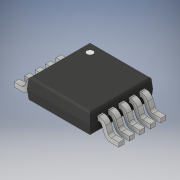
# Autodesk Inventor part: Semiconductor_TSOP-10
Saved by Autodesk Inventor 2017 (Build 210142000, 142)
## iProperties
Created: 2016-07-22
Part Number: Semiconductor_TSOP-10
Material: ABS Plastic
Document SubType Name: Modeling
Designer: Bradley
Density: 1.06 g/cm^3
Appearance: Smooth - Black
Mass: 0.00993513 g
Surface Area: 0.40182 cm^2
Volume: 0.00937276 cm^3
Author: Bradley
Autodesk Inventor part; units mm, degrees
ref_plane "YZ Plane" through (0, 0, 0) normal (1, 0, 0) x (0, 1, 0)
ref_plane "XZ Plane" through (0, 0, 0) normal (0, 1, 0) x (-1, 0, 0)
ref_plane "XY Plane" through (0, 0, 0) normal (0, 0, 1) x (1, 0, 0)
sketch "Sketch1" plane through (0, 0, 0) normal (0, 1, 0) x (-1, 0, 0)
  line L0 (-1.5, 1.5) -> (1.5, 1.5)
  line L1 (1.5, 1.5) -> (1.5, -1.5)
  line L2 (1.5, -1.5) -> (-1.5, -1.5)
  line L3 (-1.5, -1.5) -> (-1.5, 1.5)
  line L4 (-1.5, 1.5) -> (1.5, -1.5) construction
  line L5 (1.5, 1.5) -> (-1.5, -1.5) construction
  point P0 (0, 0)
  dimension "d0" = 3
  dimension "d1" = 3
  constraints: 12 end point, 2 midpoint, 2 parallel, 1 horizontal, 1 perpendicular
  measures "d0" distance of L1.end L2.end
  measures "d1" distance of L0.end L1.end
extrude "Extrusion1" add sketch "Sketch1" along normal blind 0.5 draft -5
sketch "Sketch2" plane through (0, 0, 0) normal (0, -1, 0) x (1, 0, 0)
  line L0 (1.5, 1.5) -> (-1.5, 1.5) projected
  line L1 (1.5, 1.5) -> (-1.5, 1.5) projected
  line L2 (-1.5, 1.5) -> (-1.5, -1.5) projected
  line L3 (-1.5, -1.5) -> (1.5, -1.5) projected
  line L4 (1.5, -1.5) -> (1.5, 1.5) projected
  point P0 (0, 0)
extrude "Extrusion2" add sketch "Sketch2" along normal blind 0.5 draft -5
fillet "Fillet1" radius 0.1 8 edges at (-1.4563, 0.5, 0) (0, 0.5, 1.4563) (0, 0.5, -1.4563) (1.4563, 0.5, 0) (1.4563, -0.5, 0) (0, -0.5, 1.4563) (-1.4563, -0.5, 0) (0, -0.5, -1.4563)
sketch "Sketch3" plane through (0, 0, 0) normal (0, 1, 0) x (-1, 0, 0)
  line L0 (1.5, 1.5) -> (1.5, -1.5) projected
  line L1 (-1.5, 1.5) -> (1.5, 1.5) projected
  line L2 (1.5, 1.125) -> (1.55, 1.125)
  line L3 (1.55, 1.125) -> (1.55, 0.875)
  line L4 (1.55, 0.875) -> (1.5, 0.875)
  line L5 (1.5, 0.875) -> (1.5, 1.125)
  line L6 (-1.5, -1.5) -> (-1.5, 1.5) projected
  line L7 (-1.5, 1.125) -> (-1.55, 1.125)
  line L8 (-1.55, 1.125) -> (-1.55, 0.875)
  line L9 (-1.55, 0.875) -> (-1.5, 0.875)
  line L10 (-1.5, 0.875) -> (-1.5, 1.125)
  line L11 (-1.5, 0.875) -> (1.5, 0.875)
  line L12 (1.5, 0.875) -> (1.5, 1.125)
  line L13 (1.5, 1.125) -> (-1.5, 1.125)
  line L14 (-1.5, 1.125) -> (-1.5, 0.875)
  point P0 (0, 0)
  point P1 (1.5, 1)
  dimension "d7" = 0.25
  dimension "d8" = 1
  dimension "d9" = 0.05
  constraints: 24 end point, 6 parallel, 4 point on line, 3 horizontal, 3 perpendicular, 1 collinear, 1 midpoint
  measures "d7" distance of L2.end L3.end
  measures "d8" vertical distance of point (1.5, 1) point (0, 0)
  measures "d9" distance of L3.end L4.end
extrude "Extrusion3" add sketch "Sketch3" along normal blind 0.2 contours L2 L3 L4 L0 | L0 L11 L6 L13 | L6 L9 L8 L7
sketch "Sketch4" plane through (-1.55, 0, 1.125) normal (0, 0, 1) x (1, 0, 0)
  line L0 (0.0675, 0.2) -> (0.05, 0) projected
  line L1 (0, 0.2) -> (0.0675, 0.2) projected
  line L2 (0, 0) -> (0, 0.2) projected
  line L3 (0, 0) -> (0.05, 0) projected
  line L4 (3.05, 0) -> (3.0325, 0.2) projected
  line L5 (3.05, 0) -> (3.1, 0) projected
  line L6 (3.1, 0) -> (3.1, 0.2) projected
  line L7 (3.0325, 0.2) -> (3.1, 0.2) projected
  line L8 (0, 0) -> (0.05, 0) projected
  arc A0 (0, 0) -> (-0.1397, -0.0954) centre (0, -0.15) ccw
  arc A1 (-0.576, -0.6) -> (-0.25, -0.3775) centre (-0.576, -0.25) ccw
  line L9 (0, 0.2) -> (0.0675, 0.2) projected
  arc A2 (0, 0.2) -> (-0.326, -0.0225) centre (0, -0.15) ccw
  arc A3 (-0.576, -0.4) -> (-0.4363, -0.3046) centre (-0.576, -0.25) ccw
  line L10 (-0.576, -0.6) -> (-0.95, -0.6)
  line L11 (-0.95, -0.6) -> (-0.95, -0.4)
  line L12 (-0.95, -0.4) -> (-0.576, -0.4)
  line L13 (-0.326, -0.0225) -> (-0.4363, -0.3046)
  line L14 (-0.1397, -0.0954) -> (-0.25, -0.3775)
  line L15 (2.9146, -0.5) -> (0.1854, -0.5) projected
  line L16 (0, 0.2) -> (0, 0)
  line L17 (0.1854, 0.5) -> (2.9146, 0.5) projected
  line L18 (1.55, 0.5) -> (1.55, -0.5)
  line L19 (3.1, 0) -> (3.1, 0.2)
  arc A4 (3.2397, -0.0954) -> (3.1, 0) centre (3.1, -0.15) ccw
  arc A5 (3.35, -0.3775) -> (3.676, -0.6) centre (3.676, -0.25) ccw
  arc A6 (3.426, -0.0225) -> (3.1, 0.2) centre (3.1, -0.15) ccw
  arc A7 (3.5363, -0.3046) -> (3.676, -0.4) centre (3.676, -0.25) ccw
  line L20 (3.676, -0.6) -> (4.05, -0.6)
  line L21 (4.05, -0.6) -> (4.05, -0.4)
  line L22 (4.05, -0.4) -> (3.676, -0.4)
  line L23 (3.426, -0.0225) -> (3.5363, -0.3046)
  line L24 (3.2397, -0.0954) -> (3.35, -0.3775)
  point P0 (1.55, 0)
  dimension "d12" = 0.15
  dimension "d13" = 0.15
  dimension "d16" = 0.7
  dimension "d17" = 0.1
  dimension "d25" = 5
  constraints: 26 end point, 16 point on circle, 12 symmetric about line, 8 centre point, 6 tangent, 4 coincident, 2 equal length, 2 midpoint, 2 perpendicular, 1 horizontal, 1 parallel, 4 other
  measures "d12" radius of A0
  measures "d13" radius of A3
  measures "d16" distance from line of L11 L14.end
  measures "d17" distance between parallel lines of L10 L15
  measures "d25" distance between parallel lines of L21 L11
extrude "Extrusion4" add sketch "Sketch4" against normal up to surface (0.25 mm away) contours L2 A0 L14 A1 L10 L11 L12 A3 L13 A2 | L6 A6 L23 A7 L22 L21 L20 A5 L24 A4
pattern_linear "Rectangular Pattern1" count 5 spacing 0.5 along (0, 0, -1) of "Extrusion4", "Extrusion3"
sketch "Sketch5" plane through (0, 0.5, 0) normal (0, 1, 0) x (1, 0, 0)
  line L0 (1.3646, -1.3646) -> (-1.3646, -1.3646) projected
  line L1 (1.3646, 1.3646) -> (1.3646, -1.3646) projected
  line L2 (-1.3646, 1.3646) -> (1.3646, 1.3646) projected
  line L3 (-1.3646, -1.3646) -> (-1.3646, 1.3646) projected
  circle A0 centre (-1, 1) radius 0.15
  circle A1 centre (-1, 1) radius 0.3646 construction
  line L4 (-1.3646, -1.3646) -> (-1.3646, 1.3646) projected
  line L5 (-1.3646, -1.3646) -> (1.3646, -1.3646) construction
  line L6 (-1.3646, 1.3646) -> (1.3646, 1.3646) construction
  line L7 (-1.5, 1.5) -> (1.5, 1.5) projected
  point P0 (0, 0)
  dimension "d26" = 0.5
  dimension "d27" = 0.3
  constraints: 2 centre point, 2 tangent, 1 coincident
  measures "d26" distance from line of A0.centre L7
  measures "d27" diameter of A0
extrude "Extrusion5" add sketch "Sketch5" along normal blind 0.01 and the other way blind 0.255 contours A0
equation "\"d13\" = d12"
body "Solid1"
